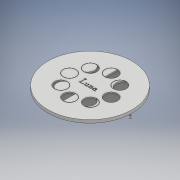
# Autodesk Inventor part: Gear Container Lid V2
Saved by Autodesk Inventor 2017 (Build 210142000, 142)
## iProperties
Created: 2019-01-21
Part Number: Gear Container Lid V2
Material: Generic
Document SubType Name: Modeling
Designer: Matt
Density: 1 g/cm^3
Appearance: Default
Author: Matt
Autodesk Inventor part; units mm, degrees
ref_plane "YZ Plane" through (0, 0, 0) normal (1, 0, 0) x (0, 1, 0)
ref_plane "XZ Plane" through (0, 0, 0) normal (0, 1, 0) x (-1, 0, 0)
ref_plane "XY Plane" through (0, 0, 0) normal (0, 0, 1) x (1, 0, 0)
sketch "Sketch1" plane through (0, 0, 0) normal (0, 0, 1) x (1, 0, 0)
  circle A0 centre (0, 0) radius 68.25
  dimension "d0" = 136.5
  constraints: 1 centre point, 1 coincident
  measures "d0" diameter of A0
extrude "Extrusion1" add sketch "Sketch1" along normal blind 5
sketch "Sketch2" plane through (0, 0, 0) normal (0, 0, -1) x (-1, 0, 0)
  circle A0 centre (0, 0) radius 68.25 projected
  line L0 (-68.25, 0) -> (-65.75, 0)
  circle A1 centre (-65.75, 0) radius 1
  line L1 (0, 0) -> (0, 3.2769)
  circle A2 centre (65.75, 0) radius 1
  dimension "d3" = 2.5
  dimension "d4" = 2
  constraints: 4 end point, 2 centre point, 1 coincident, 1 horizontal, 1 horizontal alignment, 1 symmetric about line, 1 vertical, 2 other
  measures "d3" distance of L0.start L0.end
  measures "d4" diameter of A1
extrude "Extrusion2" add sketch "Sketch2" along normal blind 4 contours A1 | A2
sketch "Sketch3" plane through (65.75, 0, -4) normal (0, 0, -1) x (-1, 0, 0)
  circle A0 centre (0, 0) radius 1.5
  line L0 (65.75, 0) -> (65.75, 4.2314)
  circle A1 centre (131.5, 0) radius 1.5
  dimension "d7" = 3
  constraints: 2 centre point, 2 end point, 1 symmetric about line, 1 vertical, 1 other
  measures "d7" diameter of A0
extrude "Extrusion3" add sketch "Sketch3" along normal blind 4
sketch "Sketch4" plane through (0, 0, 5) normal (0, 0, 1) x (1, 0, 0)
  line L0 (-14.5335, 6.1313) -> (14.7606, 6.1313) construction
  line L1 (14.7606, 6.1313) -> (14.7606, -4.9363) construction
  line L2 (14.7606, -4.9363) -> (-14.5335, -4.9363) construction
  line L3 (-14.5335, -4.9363) -> (-14.5335, 6.1313) construction
  circle A0 centre (0, 0) radius 68.25 projected
  spline S0 degree 2 poles (-8.9283, -3.3135) (-8.6738, -3.3135) (-8.296, -3.0745) (-8.1418, -2.2573) (-7.9337, -2.0876) (-7.7949, -2.0876) knots 0 0 0 1 2 3 4 4 4
  spline S1 degree 2 poles (-7.7949, -2.0876) (-7.6869, -2.0876) (-7.4711, -2.3035) (-7.4711, -2.4886) knots 0 0 0 1 2 2 2
  spline S2 degree 2 poles (-7.4711, -2.4886) (-7.4711, -3.09) (-7.3863, -3.6836) knots 0 0 0 1 1 1
  spline S3 degree 2 poles (-7.3863, -3.6836) (-7.3863, -4.0537) (-7.7409, -4.0229) knots 0 0 0 1 1 1
  spline S4 degree 2 poles (-7.7409, -4.0229) (-7.9722, -3.992) (-8.4657, -3.992) knots 0 0 0 1 1 1
  line L4 (-8.4657, -3.992) -> (-13.8011, -3.992)
  spline S5 degree 2 poles (-13.8011, -3.992) (-14.4333, -3.992) (-14.4333, -3.6682) knots 0 0 0 1 1 1
  spline S6 degree 2 poles (-14.4333, -3.6682) (-14.4333, -3.4523) (-14.2097, -3.3367) (-13.9707, -3.329) knots 0 0 0 1 2 2 2
  spline S7 degree 2 poles (-13.9707, -3.329) (-13.5235, -3.2981) (-13.3076, -2.8818) (-13.3076, -2.6119) knots 0 0 0 1 2 2 2
  line L5 (-13.3076, -2.6119) -> (-13.3076, 4.5816)
  spline S8 degree 2 poles (-13.3076, 4.5816) (-13.3076, 4.836) (-13.5543, 5.237) (-14.387, 5.4991) (-14.5566, 5.7227) (-14.5566, 5.8615) knots 0 0 0 1 2 3 4 4 4
  spline S9 degree 2 poles (-14.5566, 5.8615) (-14.5566, 5.9463) (-14.3485, 6.1005) (-14.2097, 6.1005) knots 0 0 0 1 2 2 2
  spline S10 degree 2 poles (-14.2097, 6.1005) (-14.1095, 6.1005) (-13.377, 5.8461) (-12.9298, 5.8461) knots 0 0 0 1 2 2 2
  spline S11 degree 2 poles (-12.9298, 5.8461) (-12.3747, 5.8461) (-11.3878, 6.1313) (-11.249, 6.1313) knots 0 0 0 1 2 2 2
  spline S12 degree 2 poles (-11.249, 6.1313) (-11.0871, 6.1313) (-10.8481, 5.9077) (-10.8481, 5.769) knots 0 0 0 1 2 2 2
  spline S13 degree 2 poles (-10.8481, 5.769) (-10.8481, 5.6533) (-10.9946, 5.4991) (-11.2953, 5.4374) knots 0 0 0 1 2 2 2
  spline S14 degree 2 poles (-11.2953, 5.4374) (-11.6808, 5.3603) (-11.835, 5.2292) knots 0 0 0 1 1 1
  spline S15 degree 2 poles (-11.835, 5.2292) (-12.1048, 5.0057) (-12.1048, 4.4659) knots 0 0 0 1 1 1
  line L6 (-12.1048, 4.4659) -> (-12.1048, -2.4038)
  spline S16 degree 2 poles (-12.1048, -2.4038) (-12.1048, -2.9126) (-11.781, -3.3135) (-11.4726, -3.3135) knots 0 0 0 1 2 2 2
  line L7 (-11.4726, -3.3135) -> (-8.9283, -3.3135)
  spline S17 degree 2 poles (-4.9961, -2.7199) (-4.9961, -3.0514) (-4.4873, -3.4909) (-4.1326, -3.4909) knots 0 0 0 1 2 2 2
  spline S18 degree 2 poles (-4.1326, -3.4909) (-3.909, -3.4909) (-3.3153, -3.1439) (-3.1842, -3.1439) knots 0 0 0 1 2 2 2
  spline S19 degree 2 poles (-3.1842, -3.1439) (-3.0455, -3.1439) (-3.0455, -3.3135) knots 0 0 0 1 1 1
  spline S20 degree 2 poles (-3.0455, -3.3135) (-3.0455, -3.5063) (-4.0632, -4.0923) (-4.7108, -4.0923) knots 0 0 0 1 2 2 2
  spline S21 degree 2 poles (-4.7108, -4.0923) (-5.2043, -4.0923) (-5.9522, -3.4755) (-6.0678, -2.7199) (-6.0678, -0.2758) knots 0 0 0 1 2 3 3 3
  spline S22 degree 2 poles (-6.0678, -0.2758) (-6.0678, 0.0481) (-6.7386, 0.2023) knots 0 0 0 1 1 1
  spline S23 degree 2 poles (-6.7386, 0.2023) (-7.0316, 0.2639) (-7.0316, 0.4336) knots 0 0 0 1 1 1
  spline S24 degree 2 poles (-7.0316, 0.4336) (-7.0316, 0.5415) (-6.8465, 0.6649) (-6.7078, 0.6649) knots 0 0 0 1 2 2 2
  spline S25 degree 2 poles (-6.7078, 0.6649) (-6.6692, 0.6649) (-5.9522, 0.5569) (-5.7054, 0.5569) knots 0 0 0 1 2 2 2
  spline S26 degree 2 poles (-5.7054, 0.5569) (-5.6129, 0.5569) (-5.266, 0.6572) (-5.2197, 0.6572) knots 0 0 0 1 2 2 2
  spline S27 degree 2 poles (-5.2197, 0.6572) (-4.9961, 0.6572) (-4.9961, -0.2758) knots 0 0 0 1 1 1
  line L8 (-4.9961, -0.2758) -> (-4.9961, -2.7199)
  spline S28 degree 2 poles (-2.7371, -0.376) (-2.7371, 0.1174) (-3.2691, 0.1945) knots 0 0 0 1 1 1
  spline S29 degree 2 poles (-3.2691, 0.1945) (-3.5929, 0.2408) (-3.7548, 0.3873) (-3.7548, 0.503) knots 0 0 0 1 2 2 2
  spline S30 degree 2 poles (-3.7548, 0.503) (-3.7548, 0.7574) (-3.3616, 0.7574) knots 0 0 0 1 1 1
  spline S31 degree 2 poles (-3.3616, 0.7574) (-3.2613, 0.7574) (-2.6368, 0.6109) (-2.2745, 0.6109) knots 0 0 0 1 2 2 2
  spline S32 degree 2 poles (-2.2745, 0.6109) (-2.1819, 0.6109) (-1.8967, 0.6649) (-1.8581, 0.6649) knots 0 0 0 1 2 2 2
  spline S33 degree 2 poles (-1.8581, 0.6649) (-1.6731, 0.6649) (-1.6731, 0.2485) knots 0 0 0 1 1 1
  spline S34 degree 2 poles (-1.6731, 0.2485) (-1.6731, -2.9049) (-1.5651, -3.3058) (-1.064, -3.4292) knots 0 0 0 1 2 2 2
  spline S35 degree 2 poles (-1.064, -3.4292) (-0.8018, -3.4986) (-0.6785, -3.6065) (-0.6785, -3.6836) knots 0 0 0 1 2 2 2
  spline S36 degree 2 poles (-0.6785, -3.6836) (-0.6785, -3.7762) (-0.9021, -3.9304) (-1.0871, -3.9304) knots 0 0 0 1 2 2 2
  spline S37 degree 2 poles (-1.0871, -3.9304) (-1.1642, -3.9304) (-1.7502, -3.8378) (-1.8735, -3.8378) knots 0 0 0 1 2 2 2
  spline S38 degree 2 poles (-1.8735, -3.8378) (-2.0046, -3.8378) (-2.3824, -3.9304) (-2.4441, -3.9304) knots 0 0 0 1 2 2 2
  spline S39 degree 2 poles (-2.4441, -3.9304) (-2.5906, -3.9304) (-2.7062, -3.7684) (-2.7371, -3.1208) (-2.7371, -2.2033) knots 0 0 0 1 2 3 3 3
  line L9 (-2.7371, -2.2033) -> (-2.7371, -0.376)
  spline S40 degree 2 poles (5.0501, -2.928) (5.0501, -3.221) (5.2506, -3.4061) (5.7595, -3.5217) (5.7595, -3.6836) knots 0 0 0 1 2 3 3 3
  spline S41 degree 2 poles (5.7595, -3.6836) (5.7595, -3.8995) (5.505, -3.8995) knots 0 0 0 1 1 1
  spline S42 degree 2 poles (5.505, -3.8995) (5.4588, -3.8995) (4.734, -3.8533) (4.4873, -3.8533) knots 0 0 0 1 2 2 2
  spline S43 degree 2 poles (4.4873, -3.8533) (4.071, -3.8533) (3.5081, -3.9535) (3.431, -3.9535) knots 0 0 0 1 2 2 2
  spline S44 degree 2 poles (3.431, -3.9535) (3.3077, -3.9535) (3.0918, -3.7839) (3.0918, -3.6682) knots 0 0 0 1 2 2 2
  spline S45 degree 2 poles (3.0918, -3.6682) (3.0918, -3.5834) (3.2691, -3.4215) (3.3848, -3.4215) knots 0 0 0 1 2 2 2
  spline S46 degree 2 poles (3.3848, -3.4215) (3.6084, -3.4215) (3.9476, -3.1671) (3.9476, -2.9126) knots 0 0 0 1 2 2 2
  spline S47 degree 2 poles (3.9476, -2.9126) (3.9476, -1.2627) (3.9861, -0.4762) (3.9861, -0.43) knots 0 0 0 1 2 2 2
  spline S48 degree 2 poles (3.9861, -0.43) (3.9861, 0.102) (3.5004, 0.102) knots 0 0 0 1 1 1
  spline S49 degree 2 poles (3.5004, 0.102) (3.2845, 0.102) (2.5058, -0.5456) (2.3439, -0.5456) knots 0 0 0 1 2 2 2
  spline S50 degree 2 poles (2.3439, -0.5456) (2.2899, -0.5456) (2.1511, -0.4068) (2.1511, -0.3297) knots 0 0 0 1 2 2 2
  spline S51 degree 2 poles (2.1511, -0.3297) (2.1511, -0.0907) (3.4079, 0.9039) (4.0093, 0.9039) knots 0 0 0 1 2 2 2
  spline S52 degree 2 poles (4.0093, 0.9039) (4.3639, 0.9039) (4.8882, 0.5415) (5.0579, -0.0059) (5.0579, -0.5071) knots 0 0 0 1 2 3 3 3
  line L10 (5.0579, -0.5071) -> (5.0501, -0.9465)
  line L11 (5.0501, -0.9465) -> (5.0501, -2.928)
  spline S53 degree 2 poles (0.8481, -0.2835) (0.8481, -0.029) (0.6477, 0.2254) (0.0232, 0.3333) (0.0232, 0.5569) knots 0 0 0 1 2 3 3 3
  spline S54 degree 2 poles (0.0232, 0.5569) (0.0232, 0.6572) (0.2467, 0.8422) (0.4241, 0.8422) knots 0 0 0 1 2 2 2
  spline S55 degree 2 poles (0.4241, 0.8422) (0.4935, 0.8422) (0.8713, 0.742) (1.0023, 0.742) knots 0 0 0 1 2 2 2
  spline S56 degree 2 poles (1.0023, 0.742) (1.0717, 0.742) (1.6191, 0.8268) (1.6885, 0.8268) knots 0 0 0 1 2 2 2
  spline S57 degree 2 poles (1.6885, 0.8268) (1.8196, 0.8268) (1.9353, 0.6032) (1.943, 0.2562) knots 0 0 0 1 2 2 2
  spline S58 degree 2 poles (1.943, 0.2562) (1.9507, -0.3143) (1.9507, -0.9543) knots 0 0 0 1 1 1
  line L12 (1.9507, -0.9543) -> (1.9121, -2.9126)
  spline S59 degree 2 poles (1.9121, -2.9126) (1.9121, -3.1208) (1.9815, -3.221) (2.236, -3.3675) (2.6369, -3.4523) (2.7448, -3.5988) (2.7448, -3.6913) knots 0 0 0 1 2 3 4 5 5 5
  spline S60 degree 2 poles (2.7448, -3.6913) (2.7448, -3.9226) (2.3902, -3.9226) knots 0 0 0 1 1 1
  spline S61 degree 2 poles (2.3902, -3.9226) (2.1357, -3.9226) (1.6191, -3.8378) (1.3647, -3.8378) knots 0 0 0 1 2 2 2
  spline S62 degree 2 poles (1.3647, -3.8378) (1.1565, -3.8378) (0.5012, -3.9072) (0.347, -3.9072) knots 0 0 0 1 2 2 2
  spline S63 degree 2 poles (0.347, -3.9072) (-0.0077, -3.9072) (-0.0077, -3.6528) knots 0 0 0 1 1 1
  spline S64 degree 2 poles (-0.0077, -3.6528) (-0.0077, -3.5449) (0.1157, -3.4061) (0.3239, -3.3906) knots 0 0 0 1 2 2 2
  spline S65 degree 2 poles (0.3239, -3.3906) (0.5552, -3.3752) (0.6091, -3.3213) knots 0 0 0 1 1 1
  spline S66 degree 2 poles (0.6091, -3.3213) (0.7633, -3.1593) (0.8481, -2.9126) (0.8481, -2.5271) knots 0 0 0 1 2 2 2
  line L13 (0.8481, -2.5271) -> (0.8481, -0.2835)
  spline S67 degree 2 poles (11.4418, -2.7044) (11.4418, -3.1979) (12.0972, -3.3906) knots 0 0 0 1 1 1
  spline S68 degree 2 poles (12.0972, -3.3906) (12.2668, -3.4369) (12.421, -3.568) (12.421, -3.7376) knots 0 0 0 1 2 2 2
  spline S69 degree 2 poles (12.421, -3.7376) (12.421, -3.8301) (12.2051, -3.9612) (12.0818, -3.9612) knots 0 0 0 1 2 2 2
  spline S70 degree 2 poles (12.0818, -3.9612) (11.9584, -3.9612) (11.5112, -3.8378) (11.3724, -3.8378) knots 0 0 0 1 2 2 2
  spline S71 degree 2 poles (11.3724, -3.8378) (11.2105, -3.8378) (10.7325, -3.9612) (10.6554, -3.9612) knots 0 0 0 1 2 2 2
  spline S72 degree 2 poles (10.6554, -3.9612) (10.5552, -3.9612) (10.3701, -3.8224) (10.3701, -3.753) knots 0 0 0 1 2 2 2
  spline S73 degree 2 poles (10.3701, -3.753) (10.3701, -3.6451) (10.3007, -3.6451) knots 0 0 0 1 1 1
  spline S74 degree 2 poles (10.3007, -3.6451) (10.2545, -3.6451) (10.1774, -3.6913) knots 0 0 0 1 1 1
  spline S75 degree 2 poles (10.1774, -3.6913) (9.4063, -4.1771) (8.5043, -4.1771) knots 0 0 0 1 1 1
  spline S76 degree 2 poles (8.5043, -4.1771) (8.0802, -4.1771) (7.0316, -3.7376) (6.3994, -2.8201) (6.3994, -2.1493) knots 0 0 0 1 2 3 3 3
  spline S77 degree 2 poles (6.3994, -2.1493) (6.3994, -1.44) (7.7641, -0.3374) (8.8358, -0.3374) knots 0 0 0 1 2 2 2
  spline S78 degree 2 poles (8.8358, -0.3374) (9.1982, -0.3374) (10.0694, -0.7384) (10.0694, -0.9543) knots 0 0 0 1 2 2 2
  spline S79 degree 2 poles (10.0694, -0.9543) (10.0694, -1.0545) (9.8921, -1.1778) (9.761, -1.1778) knots 0 0 0 1 2 2 2
  spline S80 degree 2 poles (9.761, -1.1778) (9.6685, -1.1778) (9.1519, -0.9311) (8.8744, -0.9311) knots 0 0 0 1 2 2 2
  spline S81 degree 2 poles (8.8744, -0.9311) (8.3115, -0.9311) (7.5713, -1.5942) (7.5713, -2.1493) knots 0 0 0 1 2 2 2
  spline S82 degree 2 poles (7.5713, -2.1493) (7.5713, -2.797) (8.4195, -3.4909) (8.9823, -3.4909) knots 0 0 0 1 2 2 2
  spline S83 degree 2 poles (8.9823, -3.4909) (9.4834, -3.4909) (10.3239, -2.8355) (10.3239, -2.2804) knots 0 0 0 1 2 2 2
  line L14 (10.3239, -2.2804) -> (10.3239, -0.4223)
  spline S84 degree 2 poles (10.3239, -0.4223) (10.3239, -0.0059) (9.7687, 0.5184) (9.3061, 0.5184) knots 0 0 0 1 2 2 2
  spline S85 degree 2 poles (9.3061, 0.5184) (8.7047, 0.5184) (8.1419, 0.1406) knots 0 0 0 1 1 1
  spline S86 degree 2 poles (8.1419, 0.1406) (7.9491, 0.0095) (7.8875, 0.0095) knots 0 0 0 1 1 1
  spline S87 degree 2 poles (7.8875, 0.0095) (7.7178, 0.0095) (7.4865, 0.1791) (7.4865, 0.3179) knots 0 0 0 1 2 2 2
  spline S88 degree 2 poles (7.4865, 0.3179) (7.4865, 0.6572) (8.7124, 1.1198) (9.4449, 1.1198) knots 0 0 0 1 2 2 2
  spline S89 degree 2 poles (9.4449, 1.1198) (10.347, 1.1198) (11.4418, 0.2177) (11.4418, -0.4068) knots 0 0 0 1 2 2 2
  line L15 (11.4418, -0.4068) -> (11.4418, -2.7044)
  constraints: 2 other
emboss "Emboss1" sketch "Sketch4" operation cut depth 2 direction (0, 0, -1) contours S0 S1 S2 S3 S4 L4 S5 S6 S7 L5 S8 S9 S10 S11 S12 S13 S14 S15 L6 S16 L7 | S17 S18 S19 S20 S21 S22 S23 S24 S25 S26 S27 L8 | S28 S29 S30 S31 S32 S33 S34 S35 S36 S37 S38 S39 L9 | S40 S41 S42 S43 S44 S45 S46 S47 S48 S49 S50 S51 S52 L10 L11 | S53 S54 S55 S56 S57 S58 L12 S59 S60 S61 S62 S63 S64 S65 S66 L13 | S67 S68 S69 S70 S71 S72 S73 S74 S75 S76 S77 S78 S79 S80 S81 S82 S83 L14 S84 S85 S86 S87 S88 S89 L15
sketch "Sketch5" plane through (0, 0, 5) normal (0, 0, 1) x (1, 0, 0)
  line L0 (0.0232, 0.5569) -> (0.0232, 68.25)
  circle A0 centre (0, 0) radius 68.25 projected
  circle A1 centre (0.0232, 34.4035) radius 10
  circle A2 centre (-23.91, 24.49) radius 10
  circle A3 centre (-33.8234, 0.5569) radius 10
  circle A4 centre (-23.91, -23.3762) radius 10
  circle A5 centre (0.0232, -33.2896) radius 10
  circle A6 centre (23.9563, -23.3762) radius 10
  circle A7 centre (33.8697, 0.5569) radius 10
  circle A8 centre (23.9563, 24.49) radius 10
  arc A9 (23.9563, 34.49) -> (23.9563, 14.49) centre (28.5388, 24.49) ccw
  arc A10 (-23.91, 14.49) -> (-23.91, 34.49) centre (-28.4925, 24.49) ccw
  arc A11 (-23.91, -13.3762) -> (-23.91, -33.3762) centre (-19.3274, -23.3762) ccw
  line L1 (0.0232, 24.4035) -> (0.0232, 44.4035)
  line L2 (0.0232, -23.2896) -> (0.0232, -43.2896)
  arc A12 (25.2693, -33.2896) -> (23.9563, -13.3762) centre (19.9933, -23.6375) ccw
  circle A13 centre (0.0232, 34.4035) radius 10.5
  circle A14 centre (-23.91, 24.49) radius 10.5
  circle A15 centre (-33.8234, 0.5569) radius 10.5
  circle A16 centre (-23.91, -23.3762) radius 10.5
  circle A17 centre (0.0232, -33.2896) radius 10.5
  circle A18 centre (23.9563, -23.3762) radius 10.5
  circle A19 centre (33.8697, 0.5569) radius 10.5
  circle A20 centre (23.9563, 24.49) radius 10.5
  dimension "d19" = 20
  dimension "d22" = 360
  dimension "d24" = 11
  dimension "d25" = 11
  dimension "d26" = 11
  dimension "d27" = 11
  dimension "d28" = 0.5
  dimension "d31" = 360
  constraints: 20 centre point, 20 point on circle, 6 end point, 2 point on line, 2 vertical, 1 midpoint, 36 other
  measures "d19" diameter of A1
  measures "d24" radius of A9
  measures "d25" radius of A10
  measures "d26" radius of A11
  measures "d27" radius of A12
  measures "d28" radial gap between concentric circles of A1 A13
emboss "Emboss2" sketch "Sketch5" operation cut depth 2 direction (0, 0, -1) picked at (2.6293, 32.3252) picked at (-16.477, 26.0613) picked at (-31.4022, -22.1449) picked at (-2.3236, -30.2412) picked at (25.1968, -21.6925) picked at (23.0228, 22.9187) contours A1 L0 A13 | L0 A13 A1 | L0 A1 | A2 A10 | A11 A4 | L2 A5 | A12 A6 | A7 | A8 A9 | A14 | A15 | A16 | A17 | A18 | A19 | A20
body "Solid1"
